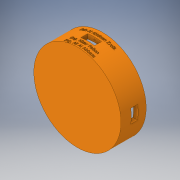
# Autodesk Inventor part: Base
Saved by Autodesk Inventor 2019 (Build 230136000, 136)
## iProperties
Created: 2022-07-05
Part Number: Base
Material: Generic
Document SubType Name: Modeling
Designer: zreik
Density: 1 g/cm^3
Appearance: Orange
Author: zreik
Autodesk Inventor part; units mm, degrees
(part 1 of 2)
ref_plane "YZ Plane" through (0, 0, 0) normal (1, 0, 0) x (0, 1, 0)
ref_plane "XY Plane" through (0, 0, 0) normal (0, 0, 1) x (1, 0, 0)
sketch "Sketch1" plane through (0, 0, 0) normal (0, 0, 1) x (1, 0, 0)
  circle A0 centre (0, 0) radius 95
  circle A1 centre (0, 0) radius 85
  circle A2 centre (0, 90) radius 1.5
  circle A3 centre (-77.9423, -45) radius 1.5
  circle A4 centre (77.9423, -45) radius 1.5
  dimension "d2" = 190
  dimension "d3" = 170
  dimension "d4" = 3
  dimension "d5" = 0
  dimension "d6" = 90
  dimension "d7" = 360
  constraints: 5 centre point, 3 coincident, 7 other
  measures "d2" diameter of A0
  measures "d3" diameter of A1
  measures "d4" diameter of A2
  measures "d5" horizontal distance of point (0, 0) A2.centre
  measures "d6" distance of point (0, 0) A2.centre
extrude "Extrusion1" add sketch "Sketch1" along normal blind 5 contours A0 | A1
extrude "Extrusion2" add sketch "Sketch1" against normal blind 50
extrude "Extrusion3" add sketch "Sketch1" along normal mid plane 10 contours A2 | A3 | A4
sketch "Sketch2" plane through (0, 0, 0) normal (0, 1, 0) x (-1, 0, 0)
  line L0 (-15, -17.5) -> (15, -17.5)
  line L1 (15, -17.5) -> (15, -32.5)
  line L2 (15, -32.5) -> (-15, -32.5)
  line L3 (-15, -32.5) -> (-15, -17.5)
  line L4 (-15, -17.5) -> (15, -32.5) construction
  line L5 (15, -17.5) -> (-15, -32.5) construction
  point P0 (0, 0)
  point P1 (0, -25)
  dimension "d14" = 0
  dimension "d15" = 25
  dimension "d16" = 30
  dimension "d17" = 15
  constraints: 12 end point, 2 midpoint, 2 parallel, 1 horizontal, 1 perpendicular
  measures "d14" horizontal distance of point (0, 0) point (0, -25)
  measures "d15" distance of point (0, 0) point (0, -25)
  measures "d16" distance of L1.end L2.end
  measures "d17" distance of L0.end L1.end
extrude "Extrusion4" cut sketch "Sketch2" against normal through all
pattern_circular "Circular Pattern1" count 4 over 360 about axis through (0, 0, 0) along (0, 0, -1) of "Extrusion4"
extrude "Extrusion5" add sketch "Sketch1" against normal blind 17.5 contours A2 | A3 | A4
ref_plane "Work Plane1" through (0, 100, 0) normal (0, 1, 0) x (-1, 0, 0)
sketch "Sketch3" plane through (0, 100, 0) normal (0, 1, 0) x (-1, 0, 0)
  line L0 (40, -45) -> (-40, -45) construction
  line L1 (-40, -45) -> (-40, -35) construction
  line L2 (-40, -35) -> (40, -35) construction
  line L3 (40, -35) -> (40, -45) construction
  line L4 (-95, -50) -> (95, -50) projected
  line L5 (40, -12.5) -> (-40, -12.5) construction
  line L6 (-40, -12.5) -> (-40, 2.5) construction
  line L7 (-40, 2.5) -> (40, 2.5) construction
  line L8 (40, 2.5) -> (40, -12.5) construction
  line L9 (95, 5) -> (-95, 5) projected
  line L10 (34.724, -36.8783) -> (38.9851, -36.8783)
  line L11 (38.9851, -36.8783) -> (38.9851, -37.6346)
  line L12 (38.9851, -37.6346) -> (35.7226, -42.2566)
  line L13 (35.7226, -42.2566) -> (38.8368, -42.2566)
  line L14 (38.8368, -42.2566) -> (38.8368, -42.9783)
  line L15 (38.8368, -42.9783) -> (34.8081, -42.9783)
  line L16 (34.8081, -42.9783) -> (34.8081, -42.2467)
  line L17 (34.8081, -42.2467) -> (38.1052, -37.6)
  line L18 (38.1052, -37.6) -> (34.724, -37.6)
  line L19 (34.724, -37.6) -> (34.724, -36.8783)
  spline S0 degree 2 poles (31.9953, -36.7745) (33.0927, -36.7745) (34.2989, -38.0054) (34.2989, -39.1423) knots 0 0 0 1 2 2 2
  spline S1 degree 2 poles (34.2989, -39.1423) (34.2989, -40.2595) (33.1274, -41.5843) (32.1832, -41.5843) knots 0 0 0 1 2 2 2
  spline S2 degree 2 poles (32.1832, -41.5843) (31.7581, -41.5843) (31.1006, -41.3372) (30.8584, -41.0752) knots 0 0 0 1 2 2 2
  spline S3 degree 2 poles (30.8584, -41.0752) (30.6112, -40.8132) (30.3492, -40.0568) (30.3492, -39.5081) knots 0 0 0 1 2 2 2
  line L20 (30.3492, -39.5081) -> (30.3492, -39.088)
  line L21 (30.3492, -39.088) -> (33.5179, -39.088)
  spline S4 degree 2 poles (33.5179, -39.088) (33.5179, -38.2921) (32.7171, -37.4468) (32.0052, -37.4468) knots 0 0 0 1 2 2 2
  spline S5 degree 2 poles (32.0052, -37.4468) (31.7531, -37.4468) (31.2637, -37.5605) (31.066, -37.6495) knots 0 0 0 1 2 2 2
  spline S6 degree 2 poles (31.066, -37.6495) (30.8584, -37.7483) (30.5717, -37.9214) (30.4778, -38.0004) knots 0 0 0 1 2 2 2
  line L22 (30.4778, -38.0004) -> (30.4333, -38.0004)
  line L23 (30.4333, -38.0004) -> (30.4333, -37.1601)
  spline S7 degree 2 poles (30.4333, -37.1601) (30.5667, -37.1057) (30.9721, -36.9475) (31.1303, -36.903) knots 0 0 0 1 2 2 2
  spline S8 degree 2 poles (31.1303, -36.903) (31.3527, -36.8388) (31.7185, -36.7745) (31.9953, -36.7745) knots 0 0 0 1 2 2 2
  spline S9 degree 2 poles (31.1006, -39.6762) (31.1105, -39.9876) (31.239, -40.4424) (31.3626, -40.5957) knots 0 0 0 1 2 2 2
  spline S10 degree 2 poles (31.3626, -40.5957) (31.4961, -40.7687) (31.9162, -40.9516) (32.2277, -40.9516) knots 0 0 0 1 2 2 2
  spline S11 degree 2 poles (32.2277, -40.9516) (32.5342, -40.9516) (32.9642, -40.7687) (33.1422, -40.5907) knots 0 0 0 1 2 2 2
  spline S12 degree 2 poles (33.1422, -40.5907) (33.3152, -40.4078) (33.4932, -39.9679) (33.5179, -39.6762) knots 0 0 0 1 2 2 2
  line L24 (33.5179, -39.6762) -> (31.1006, -39.6762)
  line L25 (28.7822, -36.8783) -> (29.5534, -36.8783)
  line L26 (29.5534, -36.8783) -> (29.5534, -41.4558)
  line L27 (29.5534, -41.4558) -> (28.7822, -41.4558)
  line L28 (28.7822, -41.4558) -> (28.7822, -36.8783)
  line L29 (28.7278, -42.2171) -> (29.6028, -42.2171)
  line L30 (29.6028, -42.2171) -> (29.6028, -43.0179)
  line L31 (29.6028, -43.0179) -> (28.7278, -43.0179)
  line L32 (28.7278, -43.0179) -> (28.7278, -42.2171)
  line L33 (24.0564, -36.8783) -> (24.8276, -36.8783)
  line L34 (24.8276, -36.8783) -> (24.8276, -39.4884)
  spline S13 degree 2 poles (24.8276, -39.4884) (24.8276, -39.8047) (24.8869, -40.3485) (24.9759, -40.5116) knots 0 0 0 1 2 2 2
  spline S14 degree 2 poles (24.9759, -40.5116) (25.0698, -40.6846) (25.406, -40.8527) (25.6927, -40.8527) knots 0 0 0 1 2 2 2
  spline S15 degree 2 poles (25.6927, -40.8527) (25.9794, -40.8527) (26.5874, -40.5462) (26.8791, -40.2991) knots 0 0 0 1 2 2 2
  line L35 (26.8791, -40.2991) -> (26.8791, -36.8783)
  line L36 (26.8791, -36.8783) -> (27.6502, -36.8783)
  line L37 (27.6502, -36.8783) -> (27.6502, -41.4558)
  line L38 (27.6502, -41.4558) -> (26.8791, -41.4558)
  line L39 (26.8791, -41.4558) -> (26.8791, -40.9466)
  spline S16 degree 2 poles (26.8791, -40.9466) (26.533, -41.2581) (25.8657, -41.5843) (25.49, -41.5843) knots 0 0 0 1 2 2 2
  spline S17 degree 2 poles (25.49, -41.5843) (24.8177, -41.5843) (24.0564, -40.6945) (24.0564, -39.8492) knots 0 0 0 1 2 2 2
  line L40 (24.0564, -39.8492) -> (24.0564, -36.8783)
  line L41 (20.9521, -36.8783) -> (18.8957, -42.9783)
  line L42 (18.8957, -42.9783) -> (17.8971, -42.9783)
  line L43 (17.8971, -42.9783) -> (15.8407, -36.8783)
  line L44 (15.8407, -36.8783) -> (16.6959, -36.8783)
  line L45 (16.6959, -36.8783) -> (17.2496, -38.5838)
  line L46 (17.2496, -38.5838) -> (19.5778, -38.5838)
  line L47 (19.5778, -38.5838) -> (20.1315, -36.8783)
  line L48 (20.1315, -36.8783) -> (20.9521, -36.8783)
  line L49 (17.472, -39.2758) -> (18.4162, -42.1479)
  line L50 (18.4162, -42.1479) -> (19.3554, -39.2758)
  line L51 (19.3554, -39.2758) -> (17.472, -39.2758)
  line L52 (14.5357, -36.8783) -> (15.3068, -36.8783)
  line L53 (15.3068, -36.8783) -> (15.3068, -43.2502)
  line L54 (15.3068, -43.2502) -> (14.5357, -43.2502)
  line L55 (14.5357, -43.2502) -> (14.5357, -36.8783)
  line L56 (11.3819, -36.8783) -> (9.3255, -42.9783)
  line L57 (9.3255, -42.9783) -> (8.3269, -42.9783)
  line L58 (8.3269, -42.9783) -> (6.2705, -36.8783)
  line L59 (6.2705, -36.8783) -> (7.1257, -36.8783)
  line L60 (7.1257, -36.8783) -> (7.6794, -38.5838)
  line L61 (7.6794, -38.5838) -> (10.0077, -38.5838)
  line L62 (10.0077, -38.5838) -> (10.5613, -36.8783)
  line L63 (10.5613, -36.8783) -> (11.3819, -36.8783)
  line L64 (7.9018, -39.2758) -> (8.846, -42.1479)
  line L65 (8.846, -42.1479) -> (9.7852, -39.2758)
  line L66 (9.7852, -39.2758) -> (7.9018, -39.2758)
  spline S18 degree 2 poles (1.9155, -39.2412) (1.9155, -38.1191) (3.003, -36.7498) (3.8236, -36.7498) knots 0 0 0 1 2 2 2
  spline S19 degree 2 poles (3.8236, -36.7498) (4.1944, -36.7498) (4.7233, -36.9327) (4.9803, -37.0909) knots 0 0 0 1 2 2 2
  line L67 (4.9803, -37.0909) -> (5.0298, -36.8783)
  line L68 (5.0298, -36.8783) -> (5.7515, -36.8783)
  line L69 (5.7515, -36.8783) -> (5.7515, -43.2502)
  line L70 (5.7515, -43.2502) -> (4.9803, -43.2502)
  line L71 (4.9803, -43.2502) -> (4.9803, -40.9763)
  spline S20 degree 2 poles (4.9803, -40.9763) (4.6887, -41.2383) (4.0115, -41.5843) (3.5814, -41.5843) knots 0 0 0 1 2 2 2
  spline S21 degree 2 poles (3.5814, -41.5843) (2.8053, -41.5843) (1.9155, -40.3436) (1.9155, -39.2412) knots 0 0 0 1 2 2 2
  spline S22 degree 2 poles (2.7114, -39.1819) (2.7114, -40.0025) (3.2107, -40.8527) (3.7643, -40.8527) knots 0 0 0 1 2 2 2
  spline S23 degree 2 poles (3.7643, -40.8527) (4.0757, -40.8527) (4.7184, -40.5561) (4.9803, -40.3287) knots 0 0 0 1 2 2 2
  line L72 (4.9803, -40.3287) -> (4.9803, -37.7038)
  spline S24 degree 2 poles (4.9803, -37.7038) (4.6887, -37.5605) (4.2389, -37.4419) (3.9719, -37.4419) knots 0 0 0 1 2 2 2
  spline S25 degree 2 poles (3.9719, -37.4419) (3.3837, -37.4419) (2.7114, -38.2773) (2.7114, -39.1819) knots 0 0 0 1 2 2 2
  line L73 (0.3287, -36.8783) -> (1.0999, -36.8783)
  line L74 (1.0999, -36.8783) -> (1.0999, -41.4558)
  line L75 (1.0999, -41.4558) -> (0.3287, -41.4558)
  line L76 (0.3287, -41.4558) -> (0.3287, -36.8783)
  line L77 (0.2744, -42.2171) -> (1.1493, -42.2171)
  line L78 (1.1493, -42.2171) -> (1.1493, -43.0179)
  line L79 (1.1493, -43.0179) -> (0.2744, -43.0179)
  line L80 (0.2744, -43.0179) -> (0.2744, -42.2171)
  line L81 (-4.3229, -36.8783) -> (-3.5517, -36.8783)
  line L82 (-3.5517, -36.8783) -> (-3.5517, -37.343)
  spline S26 degree 2 poles (-3.5517, -37.343) (-3.3738, -37.1947) (-3.1118, -36.997) (-2.9338, -36.9129) knots 0 0 0 1 2 2 2
  spline S27 degree 2 poles (-2.9338, -36.9129) (-2.7707, -36.8338) (-2.4197, -36.7498) (-2.1874, -36.7498) knots 0 0 0 1 2 2 2
  spline S28 degree 2 poles (-2.1874, -36.7498) (-1.8117, -36.7498) (-1.179, -37.0612) (-0.9565, -37.3628) knots 0 0 0 1 2 2 2
  spline S29 degree 2 poles (-0.9565, -37.3628) (-0.7341, -37.6643) (-0.4869, -38.5541) (-0.4869, -39.1325) knots 0 0 0 1 2 2 2
  spline S30 degree 2 poles (-0.4869, -39.1325) (-0.4869, -39.7355) (-0.7983, -40.6154) (-1.0702, -40.9466) knots 0 0 0 1 2 2 2
  spline S31 degree 2 poles (-1.0702, -40.9466) (-1.3223, -41.2432) (-2.0292, -41.5843) (-2.4197, -41.5843) knots 0 0 0 1 2 2 2
  spline S32 degree 2 poles (-2.4197, -41.5843) (-2.7608, -41.5843) (-3.27, -41.4311) (-3.5517, -41.2729) knots 0 0 0 1 2 2 2
  line L83 (-3.5517, -41.2729) -> (-3.5517, -43.2502)
  line L84 (-3.5517, -43.2502) -> (-4.3229, -43.2502)
  line L85 (-4.3229, -43.2502) -> (-4.3229, -36.8783)
  line L86 (-3.5517, -37.9906) -> (-3.5517, -40.6352)
  spline S33 degree 2 poles (-3.5517, -40.6352) (-3.265, -40.7736) (-2.8103, -40.8774) (-2.5483, -40.8774) knots 0 0 0 1 2 2 2
  spline S34 degree 2 poles (-2.5483, -40.8774) (-1.9551, -40.8774) (-1.2828, -39.9876) (-1.2828, -39.1473) knots 0 0 0 1 2 2 2
  spline S35 degree 2 poles (-1.2828, -39.1473) (-1.2828, -38.3366) (-1.7969, -37.4814) (-2.3654, -37.4814) knots 0 0 0 1 2 2 2
  spline S36 degree 2 poles (-2.3654, -37.4814) (-2.6669, -37.4814) (-3.2799, -37.7582) (-3.5517, -37.9906) knots 0 0 0 1 2 2 2
  spline S37 degree 2 poles (-7.4273, -36.7745) (-6.3299, -36.7745) (-5.1237, -38.0054) (-5.1237, -39.1423) knots 0 0 0 1 2 2 2
  spline S38 degree 2 poles (-5.1237, -39.1423) (-5.1237, -40.2595) (-6.2953, -41.5843) (-7.2394, -41.5843) knots 0 0 0 1 2 2 2
  spline S39 degree 2 poles (-7.2394, -41.5843) (-7.6645, -41.5843) (-8.322, -41.3372) (-8.5642, -41.0752) knots 0 0 0 1 2 2 2
  spline S40 degree 2 poles (-8.5642, -41.0752) (-8.8114, -40.8132) (-9.0734, -40.0568) (-9.0734, -39.5081) knots 0 0 0 1 2 2 2
  line L87 (-9.0734, -39.5081) -> (-9.0734, -39.088)
  line L88 (-9.0734, -39.088) -> (-5.9047, -39.088)
  spline S41 degree 2 poles (-5.9047, -39.088) (-5.9047, -38.2921) (-6.7056, -37.4468) (-7.4174, -37.4468) knots 0 0 0 1 2 2 2
  spline S42 degree 2 poles (-7.4174, -37.4468) (-7.6695, -37.4468) (-8.1589, -37.5605) (-8.3566, -37.6495) knots 0 0 0 1 2 2 2
  spline S43 degree 2 poles (-8.3566, -37.6495) (-8.5642, -37.7483) (-8.8509, -37.9214) (-8.9449, -38.0004) knots 0 0 0 1 2 2 2
  line L89 (-8.9449, -38.0004) -> (-8.9893, -38.0004)
  line L90 (-8.9893, -38.0004) -> (-8.9893, -37.1601)
  spline S44 degree 2 poles (-8.9893, -37.1601) (-8.8559, -37.1057) (-8.4505, -36.9475) (-8.2923, -36.903) knots 0 0 0 1 2 2 2
  spline S45 degree 2 poles (-8.2923, -36.903) (-8.0699, -36.8388) (-7.7041, -36.7745) (-7.4273, -36.7745) knots 0 0 0 1 2 2 2
  spline S46 degree 2 poles (-8.322, -39.6762) (-8.3121, -39.9876) (-8.1836, -40.4424) (-8.06, -40.5957) knots 0 0 0 1 2 2 2
  spline S47 degree 2 poles (-8.06, -40.5957) (-7.9265, -40.7687) (-7.5064, -40.9516) (-7.1949, -40.9516) knots 0 0 0 1 2 2 2
  spline S48 degree 2 poles (-7.1949, -40.9516) (-6.8885, -40.9516) (-6.4584, -40.7687) (-6.2804, -40.5907) knots 0 0 0 1 2 2 2
  spline S49 degree 2 poles (-6.2804, -40.5907) (-6.1074, -40.4078) (-5.9295, -39.9679) (-5.9047, -39.6762) knots 0 0 0 1 2 2 2
  line L91 (-5.9047, -39.6762) -> (-8.322, -39.6762)
  spline S50 degree 2 poles (-11.8416, -36.7745) (-10.7442, -36.7745) (-9.538, -38.0054) (-9.538, -39.1423) knots 0 0 0 1 2 2 2
  spline S51 degree 2 poles (-9.538, -39.1423) (-9.538, -40.2595) (-10.7096, -41.5843) (-11.6538, -41.5843) knots 0 0 0 1 2 2 2
  spline S52 degree 2 poles (-11.6538, -41.5843) (-12.0789, -41.5843) (-12.7363, -41.3372) (-12.9786, -41.0752) knots 0 0 0 1 2 2 2
  spline S53 degree 2 poles (-12.9786, -41.0752) (-13.2257, -40.8132) (-13.4877, -40.0568) (-13.4877, -39.5081) knots 0 0 0 1 2 2 2
  line L92 (-13.4877, -39.5081) -> (-13.4877, -39.088)
  line L93 (-13.4877, -39.088) -> (-10.3191, -39.088)
  spline S54 degree 2 poles (-10.3191, -39.088) (-10.3191, -38.2921) (-11.1199, -37.4468) (-11.8317, -37.4468) knots 0 0 0 1 2 2 2
  spline S55 degree 2 poles (-11.8317, -37.4468) (-12.0838, -37.4468) (-12.5732, -37.5605) (-12.7709, -37.6495) knots 0 0 0 1 2 2 2
  spline S56 degree 2 poles (-12.7709, -37.6495) (-12.9786, -37.7483) (-13.2653, -37.9214) (-13.3592, -38.0004) knots 0 0 0 1 2 2 2
  line L94 (-13.3592, -38.0004) -> (-13.4037, -38.0004)
  line L95 (-13.4037, -38.0004) -> (-13.4037, -37.1601)
  spline S57 degree 2 poles (-13.4037, -37.1601) (-13.2702, -37.1057) (-12.8649, -36.9475) (-12.7067, -36.903) knots 0 0 0 1 2 2 2
  spline S58 degree 2 poles (-12.7067, -36.903) (-12.4842, -36.8388) (-12.1184, -36.7745) (-11.8416, -36.7745) knots 0 0 0 1 2 2 2
  spline S59 degree 2 poles (-12.7363, -39.6762) (-12.7265, -39.9876) (-12.5979, -40.4424) (-12.4744, -40.5957) knots 0 0 0 1 2 2 2
  spline S60 degree 2 poles (-12.4744, -40.5957) (-12.3409, -40.7687) (-11.9207, -40.9516) (-11.6093, -40.9516) knots 0 0 0 1 2 2 2
  spline S61 degree 2 poles (-11.6093, -40.9516) (-11.3028, -40.9516) (-10.8727, -40.7687) (-10.6948, -40.5907) knots 0 0 0 1 2 2 2
  spline S62 degree 2 poles (-10.6948, -40.5907) (-10.5218, -40.4078) (-10.3438, -39.9679) (-10.3191, -39.6762) knots 0 0 0 1 2 2 2
  line L96 (-10.3191, -39.6762) -> (-12.7363, -39.6762)
  line L97 (-17.8625, -36.8783) -> (-17.0914, -36.8783)
  line L98 (-17.0914, -36.8783) -> (-17.0914, -39.4884)
  spline S63 degree 2 poles (-17.0914, -39.4884) (-17.0914, -39.8047) (-17.0321, -40.3485) (-16.9431, -40.5116) knots 0 0 0 1 2 2 2
  spline S64 degree 2 poles (-16.9431, -40.5116) (-16.8491, -40.6846) (-16.513, -40.8527) (-16.2263, -40.8527) knots 0 0 0 1 2 2 2
  spline S65 degree 2 poles (-16.2263, -40.8527) (-15.9396, -40.8527) (-15.3316, -40.5462) (-15.0399, -40.2991) knots 0 0 0 1 2 2 2
  line L99 (-15.0399, -40.2991) -> (-15.0399, -36.8783)
  line L100 (-15.0399, -36.8783) -> (-14.2688, -36.8783)
  line L101 (-14.2688, -36.8783) -> (-14.2688, -41.4558)
  line L102 (-14.2688, -41.4558) -> (-15.0399, -41.4558)
  line L103 (-15.0399, -41.4558) -> (-15.0399, -40.9466)
  spline S66 degree 2 poles (-15.0399, -40.9466) (-15.3859, -41.2581) (-16.0533, -41.5843) (-16.429, -41.5843) knots 0 0 0 1 2 2 2
  spline S67 degree 2 poles (-16.429, -41.5843) (-17.1013, -41.5843) (-17.8625, -40.6945) (-17.8625, -39.8492) knots 0 0 0 1 2 2 2
  line L104 (-17.8625, -39.8492) -> (-17.8625, -36.8783)
  line L105 (-25.5147, -36.8783) -> (-21.2536, -36.8783)
  line L106 (-21.2536, -36.8783) -> (-21.2536, -37.6346)
  line L107 (-21.2536, -37.6346) -> (-24.5162, -42.2566)
  line L108 (-24.5162, -42.2566) -> (-21.4019, -42.2566)
  line L109 (-21.4019, -42.2566) -> (-21.4019, -42.9783)
  line L110 (-21.4019, -42.9783) -> (-25.4307, -42.9783)
  line L111 (-25.4307, -42.9783) -> (-25.4307, -42.2467)
  line L112 (-25.4307, -42.2467) -> (-22.1335, -37.6)
  line L113 (-22.1335, -37.6) -> (-25.5147, -37.6)
  line L114 (-25.5147, -37.6) -> (-25.5147, -36.8783)
  line L115 (-28.6833, -40.6303) -> (-28.6438, -40.6303)
  spline S68 degree 2 poles (-28.6438, -40.6303) (-28.5548, -40.655) (-28.362, -40.6649) (-28.2286, -40.6649) knots 0 0 0 1 2 2 2
  spline S69 degree 2 poles (-28.2286, -40.6649) (-27.9171, -40.6649) (-27.3042, -40.393) (-27.0274, -40.1261) knots 0 0 0 1 2 2 2
  line L116 (-27.0274, -40.1261) -> (-27.0274, -36.8783)
  line L117 (-27.0274, -36.8783) -> (-26.2562, -36.8783)
  line L118 (-26.2562, -36.8783) -> (-26.2562, -41.4558)
  line L119 (-26.2562, -41.4558) -> (-27.0274, -41.4558)
  line L120 (-27.0274, -41.4558) -> (-27.0274, -40.7736)
  spline S70 degree 2 poles (-27.0274, -40.7736) (-27.4475, -41.1493) (-28.0753, -41.4558) (-28.3719, -41.4558) knots 0 0 0 1 2 2 2
  spline S71 degree 2 poles (-28.3719, -41.4558) (-28.4906, -41.4558) (-28.6092, -41.4459) (-28.6833, -41.4311) knots 0 0 0 1 2 2 2
  line L121 (-28.6833, -41.4311) -> (-28.6833, -40.6303)
  spline S72 degree 2 poles (-31.2687, -36.7745) (-30.1713, -36.7745) (-28.9651, -38.0054) (-28.9651, -39.1423) knots 0 0 0 1 2 2 2
  spline S73 degree 2 poles (-28.9651, -39.1423) (-28.9651, -40.2595) (-30.1367, -41.5843) (-31.0808, -41.5843) knots 0 0 0 1 2 2 2
  spline S74 degree 2 poles (-31.0808, -41.5843) (-31.506, -41.5843) (-32.1634, -41.3372) (-32.4056, -41.0752) knots 0 0 0 1 2 2 2
  spline S75 degree 2 poles (-32.4056, -41.0752) (-32.6528, -40.8132) (-32.9148, -40.0568) (-32.9148, -39.5081) knots 0 0 0 1 2 2 2
  line L122 (-32.9148, -39.5081) -> (-32.9148, -39.088)
  line L123 (-32.9148, -39.088) -> (-29.7462, -39.088)
  spline S76 degree 2 poles (-29.7462, -39.088) (-29.7462, -38.2921) (-30.547, -37.4468) (-31.2588, -37.4468) knots 0 0 0 1 2 2 2
  spline S77 degree 2 poles (-31.2588, -37.4468) (-31.5109, -37.4468) (-32.0003, -37.5605) (-32.198, -37.6495) knots 0 0 0 1 2 2 2
  spline S78 degree 2 poles (-32.198, -37.6495) (-32.4056, -37.7483) (-32.6923, -37.9214) (-32.7863, -38.0004) knots 0 0 0 1 2 2 2
  line L124 (-32.7863, -38.0004) -> (-32.8308, -38.0004)
  line L125 (-32.8308, -38.0004) -> (-32.8308, -37.1601)
  spline S79 degree 2 poles (-32.8308, -37.1601) (-32.6973, -37.1057) (-32.2919, -36.9475) (-32.1338, -36.903) knots 0 0 0 1 2 2 2
  spline S80 degree 2 poles (-32.1338, -36.903) (-31.9113, -36.8388) (-31.5455, -36.7745) (-31.2687, -36.7745) knots 0 0 0 1 2 2 2
  spline S81 degree 2 poles (-32.1634, -39.6762) (-32.1535, -39.9876) (-32.025, -40.4424) (-31.9014, -40.5957) knots 0 0 0 1 2 2 2
  spline S82 degree 2 poles (-31.9014, -40.5957) (-31.768, -40.7687) (-31.3478, -40.9516) (-31.0363, -40.9516) knots 0 0 0 1 2 2 2
  spline S83 degree 2 poles (-31.0363, -40.9516) (-30.7299, -40.9516) (-30.2998, -40.7687) (-30.1218, -40.5907) knots 0 0 0 1 2 2 2
  spline S84 degree 2 poles (-30.1218, -40.5907) (-29.9488, -40.4078) (-29.7709, -39.9679) (-29.7462, -39.6762) knots 0 0 0 1 2 2 2
  line L126 (-29.7462, -39.6762) -> (-32.1634, -39.6762)
  line L127 (-34.4818, -36.8783) -> (-33.7107, -36.8783)
  line L128 (-33.7107, -36.8783) -> (-33.7107, -41.4558)
  line L129 (-33.7107, -41.4558) -> (-34.4818, -41.4558)
  line L130 (-34.4818, -41.4558) -> (-34.4818, -36.8783)
  line L131 (-34.5362, -42.2171) -> (-33.6612, -42.2171)
  line L132 (-33.6612, -42.2171) -> (-33.6612, -43.0179)
  line L133 (-33.6612, -43.0179) -> (-34.5362, -43.0179)
  line L134 (-34.5362, -43.0179) -> (-34.5362, -42.2171)
  line L135 (-39.4053, -36.8783) -> (-38.3919, -36.8783)
  line L136 (-38.3919, -36.8783) -> (-36.6915, -39.088)
  line L137 (-36.6915, -39.088) -> (-36.385, -38.7914)
  line L138 (-36.385, -38.7914) -> (-36.385, -36.8783)
  line L139 (-36.385, -36.8783) -> (-35.6138, -36.8783)
  line L140 (-35.6138, -36.8783) -> (-35.6138, -43.2502)
  line L141 (-35.6138, -43.2502) -> (-36.385, -43.2502)
  line L142 (-36.385, -43.2502) -> (-36.385, -39.523)
  line L143 (-36.385, -39.523) -> (-38.1942, -41.4558)
  line L144 (-38.1942, -41.4558) -> (-39.1532, -41.4558)
  line L145 (-39.1532, -41.4558) -> (-37.2748, -39.5427)
  line L146 (-37.2748, -39.5427) -> (-39.4053, -36.8783)
  line L147 (30.542, -7.7009) -> (30.542, -13.8009)
  line L148 (30.542, -13.8009) -> (26.7258, -13.8009)
  line L149 (26.7258, -13.8009) -> (26.7258, -13.0792)
  line L150 (26.7258, -13.0792) -> (29.7313, -13.0792)
  line L151 (29.7313, -13.0792) -> (29.7313, -11.4083)
  line L152 (29.7313, -11.4083) -> (26.9285, -11.4083)
  line L153 (26.9285, -11.4083) -> (26.9285, -10.6866)
  line L154 (26.9285, -10.6866) -> (29.7313, -10.6866)
  line L155 (29.7313, -10.6866) -> (29.7313, -8.4226)
  line L156 (29.7313, -8.4226) -> (26.7258, -8.4226)
  line L157 (26.7258, -8.4226) -> (26.7258, -7.7009)
  line L158 (26.7258, -7.7009) -> (30.542, -7.7009)
  line L159 (22.3016, -7.7009) -> (23.0727, -7.7009)
  line L160 (23.0727, -7.7009) -> (23.0727, -10.3109)
  spline S85 degree 2 poles (23.0727, -10.3109) (23.0727, -10.6273) (23.1321, -11.1711) (23.221, -11.3342) knots 0 0 0 1 2 2 2
  spline S86 degree 2 poles (23.221, -11.3342) (23.315, -11.5072) (23.6511, -11.6753) (23.9378, -11.6753) knots 0 0 0 1 2 2 2
  spline S87 degree 2 poles (23.9378, -11.6753) (24.2245, -11.6753) (24.8325, -11.3688) (25.1242, -11.1216) knots 0 0 0 1 2 2 2
  line L161 (25.1242, -11.1216) -> (25.1242, -7.7009)
  line L162 (25.1242, -7.7009) -> (25.8953, -7.7009)
  line L163 (25.8953, -7.7009) -> (25.8953, -12.2783)
  line L164 (25.8953, -12.2783) -> (25.1242, -12.2783)
  line L165 (25.1242, -12.2783) -> (25.1242, -11.7692)
  spline S88 degree 2 poles (25.1242, -11.7692) (24.7782, -12.0806) (24.1108, -12.4069) (23.7351, -12.4069) knots 0 0 0 1 2 2 2
  spline S89 degree 2 poles (23.7351, -12.4069) (23.0628, -12.4069) (22.3016, -11.5171) (22.3016, -10.6718) knots 0 0 0 1 2 2 2
  line L166 (22.3016, -10.6718) -> (22.3016, -7.7009)
  spline S90 degree 2 poles (21.0559, -6.9693) (20.9768, -6.9347) (20.6752, -6.8259) (20.4825, -6.7814) knots 0 0 0 1 2 2 2
  spline S91 degree 2 poles (20.4825, -6.7814) (20.2699, -6.7271) (19.909, -6.6628) (19.6965, -6.6628) knots 0 0 0 1 2 2 2
  spline S92 degree 2 poles (19.6965, -6.6628) (19.3406, -6.6628) (18.8462, -6.8506) (18.7078, -7.0187) knots 0 0 0 1 2 2 2
  spline S93 degree 2 poles (18.7078, -7.0187) (18.5744, -7.1868) (18.4705, -7.6267) (18.4705, -7.9085) knots 0 0 0 1 2 2 2
  line L167 (18.4705, -7.9085) -> (18.4705, -8.3089)
  spline S94 degree 2 poles (18.4705, -8.3089) (18.782, -8.037) (19.3801, -7.78) (19.8299, -7.78) knots 0 0 0 1 2 2 2
  spline S95 degree 2 poles (19.8299, -7.78) (20.611, -7.78) (21.5354, -8.9416) (21.5354, -10.0341) knots 0 0 0 1 2 2 2
  spline S96 degree 2 poles (21.5354, -10.0341) (21.5354, -10.6026) (21.2141, -11.4825) (20.9471, -11.7939) knots 0 0 0 1 2 2 2
  spline S97 degree 2 poles (20.9471, -11.7939) (20.6901, -12.0856) (19.9832, -12.4069) (19.6075, -12.4069) knots 0 0 0 1 2 2 2
  spline S98 degree 2 poles (19.6075, -12.4069) (19.2516, -12.4069) (18.7325, -12.2388) (18.4705, -12.0856) knots 0 0 0 1 2 2 2
  line L168 (18.4705, -12.0856) -> (18.4261, -12.2783)
  line L169 (18.4261, -12.2783) -> (17.6994, -12.2783)
  line L170 (17.6994, -12.2783) -> (17.6994, -8.2249)
  spline S99 degree 2 poles (17.6994, -8.2249) (17.6994, -7.0583) (18.7128, -5.9707) (19.7558, -5.9707) knots 0 0 0 1 2 2 2
  spline S100 degree 2 poles (19.7558, -5.9707) (20.0919, -5.9707) (20.7939, -6.0795) (21.0954, -6.1685) knots 0 0 0 1 2 2 2
  line L171 (21.0954, -6.1685) -> (21.0954, -6.9693)
  line L172 (21.0954, -6.9693) -> (21.0559, -6.9693)
  line L173 (18.4705, -8.9416) -> (18.4705, -11.4578)
  spline S101 degree 2 poles (18.4705, -11.4578) (18.7573, -11.5962) (19.2417, -11.7148) (19.4839, -11.7148) knots 0 0 0 1 2 2 2
  spline S102 degree 2 poles (19.4839, -11.7148) (20.0672, -11.7148) (20.7395, -10.8547) (20.7395, -10.0489) knots 0 0 0 1 2 2 2
  spline S103 degree 2 poles (20.7395, -10.0489) (20.7395, -9.2877) (20.2303, -8.4918) (19.6569, -8.4918) knots 0 0 0 1 2 2 2
  spline S104 degree 2 poles (19.6569, -8.4918) (19.3554, -8.4918) (18.7227, -8.7291) (18.4705, -8.9416) knots 0 0 0 1 2 2 2
  line L174 (15.3859, -7.7009) -> (16.3647, -7.7009)
  line L175 (16.3647, -7.7009) -> (16.3647, -8.8675)
  line L176 (16.3647, -8.8675) -> (15.3859, -8.8675)
  line L177 (15.3859, -8.8675) -> (15.3859, -7.7009)
  line L178 (6.9972, -7.7009) -> (7.9068, -7.7009)
  line L179 (7.9068, -7.7009) -> (10.6058, -12.9605)
  line L180 (10.6058, -12.9605) -> (10.6058, -7.7009)
  line L181 (10.6058, -7.7009) -> (11.3621, -7.7009)
  line L182 (11.3621, -7.7009) -> (11.3621, -13.8009)
  line L183 (11.3621, -13.8009) -> (10.2103, -13.8009)
  line L184 (10.2103, -13.8009) -> (7.7535, -8.9713)
  line L185 (7.7535, -8.9713) -> (7.7535, -13.8009)
  line L186 (7.7535, -13.8009) -> (6.9972, -13.8009)
  line L187 (6.9972, -13.8009) -> (6.9972, -7.7009)
  line L188 (5.0347, -7.7009) -> (5.8059, -7.7009)
  line L189 (5.8059, -7.7009) -> (5.8059, -12.2783)
  line L190 (5.8059, -12.2783) -> (5.0347, -12.2783)
  line L191 (5.0347, -12.2783) -> (5.0347, -7.7009)
  line L192 (4.9803, -13.0396) -> (5.8553, -13.0396)
  line L193 (5.8553, -13.0396) -> (5.8553, -13.8404)
  line L194 (5.8553, -13.8404) -> (4.9803, -13.8404)
  line L195 (4.9803, -13.8404) -> (4.9803, -13.0396)
  line L196 (0.8972, -7.7009) -> (4.2586, -7.7009)
  line L197 (4.2586, -7.7009) -> (4.2586, -8.2743)
  line L198 (4.2586, -8.2743) -> (1.8661, -11.6456)
  line L199 (1.8661, -11.6456) -> (4.1598, -11.6456)
  line L200 (4.1598, -11.6456) -> (4.1598, -12.2783)
  line L201 (4.1598, -12.2783) -> (0.9417, -12.2783)
  line L202 (0.9417, -12.2783) -> (0.9417, -11.7296)
  line L203 (0.9417, -11.7296) -> (3.3441, -8.3484)
  line L204 (3.3441, -8.3484) -> (0.8972, -8.3484)
  line L205 (0.8972, -8.3484) -> (0.8972, -7.7009)
  spline S105 degree 2 poles (-2.3752, -8.1853) (-2.2813, -8.1161) (-1.965, -7.8689) (-1.8167, -7.7948) knots 0 0 0 1 2 2 2
  spline S106 degree 2 poles (-1.8167, -7.7948) (-1.614, -7.686) (-1.2333, -7.5724) (-0.8873, -7.5724) knots 0 0 0 1 2 2 2
  spline S107 degree 2 poles (-0.8873, -7.5724) (-0.6056, -7.5724) (-0.0964, -7.7849) (0.0964, -7.9777) knots 0 0 0 1 2 2 2
  spline S108 degree 2 poles (0.0964, -7.9777) (0.2793, -8.1655) (0.5017, -8.7192) (0.5017, -9.0257) knots 0 0 0 1 2 2 2
  spline S109 degree 2 poles (0.5017, -9.0257) (0.5017, -9.5002) (0.1013, -10.1725) (-0.3337, -10.3653) knots 0 0 0 1 2 2 2
  spline S110 degree 2 poles (-0.3337, -10.3653) (-0.7192, -10.5433) (-1.7672, -10.6767) (-2.3752, -10.7113) knots 0 0 0 1 2 2 2
  line L206 (-2.3752, -10.7113) -> (-2.3752, -10.8596)
  spline S111 degree 2 poles (-2.3752, -10.8596) (-2.3752, -11.1266) (-2.2121, -11.4578) (-2.0638, -11.5517) knots 0 0 0 1 2 2 2
  spline S112 degree 2 poles (-2.0638, -11.5517) (-1.9155, -11.6456) (-1.4904, -11.7049) (-1.263, -11.7049) knots 0 0 0 1 2 2 2
  spline S113 degree 2 poles (-1.263, -11.7049) (-0.9961, -11.7049) (-0.2744, -11.5467) (0.0865, -11.3935) knots 0 0 0 1 2 2 2
  line L207 (0.0865, -11.3935) -> (0.131, -11.3935)
  line L208 (0.131, -11.3935) -> (0.131, -12.1795)
  spline S114 degree 2 poles (0.131, -12.1795) (-0.0816, -12.2388) (-0.8774, -12.3871) (-1.2679, -12.3871) knots 0 0 0 1 2 2 2
  spline S115 degree 2 poles (-1.2679, -12.3871) (-1.7425, -12.3871) (-2.3901, -12.2388) (-2.6471, -12.046) knots 0 0 0 1 2 2 2
  spline S116 degree 2 poles (-2.6471, -12.046) (-2.8992, -11.8582) (-3.1464, -11.26) (-3.1464, -10.83) knots 0 0 0 1 2 2 2
  line L209 (-3.1464, -10.83) -> (-3.1464, -7.7009)
  line L210 (-3.1464, -7.7009) -> (-2.3752, -7.7009)
  line L211 (-2.3752, -7.7009) -> (-2.3752, -8.1853)
  line L212 (-2.3752, -8.8279) -> (-2.3752, -10.0984)
  spline S117 degree 2 poles (-2.3752, -10.0984) (-2.0984, -10.0736) (-1.263, -9.9896) (-1.001, -9.9105) knots 0 0 0 1 2 2 2
  spline S118 degree 2 poles (-1.001, -9.9105) (-0.6945, -9.8166) (-0.2941, -9.4261) (-0.2941, -9.0801) knots 0 0 0 1 2 2 2
  spline S119 degree 2 poles (-0.2941, -9.0801) (-0.2941, -8.6846) (-0.739, -8.2842) (-1.1641, -8.2842) knots 0 0 0 1 2 2 2
  spline S120 degree 2 poles (-1.1641, -8.2842) (-1.525, -8.2842) (-2.1182, -8.5956) (-2.3752, -8.8279) knots 0 0 0 1 2 2 2
  line L213 (-6.6561, -11.4528) -> (-6.6166, -11.4528)
  spline S121 degree 2 poles (-6.6166, -11.4528) (-6.5276, -11.4775) (-6.3348, -11.4874) (-6.2013, -11.4874) knots 0 0 0 1 2 2 2
  spline S122 degree 2 poles (-6.2013, -11.4874) (-5.8899, -11.4874) (-5.2769, -11.2155) (-5.0001, -10.9486) knots 0 0 0 1 2 2 2
  line L214 (-5.0001, -10.9486) -> (-5.0001, -7.7009)
  line L215 (-5.0001, -7.7009) -> (-4.229, -7.7009)
  line L216 (-4.229, -7.7009) -> (-4.229, -12.2783)
  line L217 (-4.229, -12.2783) -> (-5.0001, -12.2783)
  line L218 (-5.0001, -12.2783) -> (-5.0001, -11.5962)
  spline S123 degree 2 poles (-5.0001, -11.5962) (-5.4203, -11.9719) (-6.0481, -12.2783) (-6.3447, -12.2783) knots 0 0 0 1 2 2 2
  spline S124 degree 2 poles (-6.3447, -12.2783) (-6.4633, -12.2783) (-6.582, -12.2685) (-6.6561, -12.2536) knots 0 0 0 1 2 2 2
  line L219 (-6.6561, -12.2536) -> (-6.6561, -11.4528)
  line L220 (-13.5816, -13.0792) -> (-10.7442, -13.0792)
  line L221 (-10.7442, -13.0792) -> (-10.7442, -11.3589)
  line L222 (-10.7442, -11.3589) -> (-13.463, -11.3589)
  line L223 (-13.463, -11.3589) -> (-13.463, -10.6372)
  line L224 (-13.463, -10.6372) -> (-10.7442, -10.6372)
  line L225 (-10.7442, -10.6372) -> (-10.7442, -7.7009)
  line L226 (-10.7442, -7.7009) -> (-9.9335, -7.7009)
  line L227 (-9.9335, -7.7009) -> (-9.9335, -13.8009)
  line L228 (-9.9335, -13.8009) -> (-13.5816, -13.8009)
  line L229 (-13.5816, -13.8009) -> (-13.5816, -13.0792)
  spline S125 degree 2 poles (-16.7997, -8.1853) (-16.7058, -8.1161) (-16.3894, -7.8689) (-16.2411, -7.7948) knots 0 0 0 1 2 2 2
  spline S126 degree 2 poles (-16.2411, -7.7948) (-16.0385, -7.686) (-15.6578, -7.5724) (-15.3118, -7.5724) knots 0 0 0 1 2 2 2
  spline S127 degree 2 poles (-15.3118, -7.5724) (-15.03, -7.5724) (-14.5209, -7.7849) (-14.3281, -7.9777) knots 0 0 0 1 2 2 2
  spline S128 degree 2 poles (-14.3281, -7.9777) (-14.1452, -8.1655) (-13.9227, -8.7192) (-13.9227, -9.0257) knots 0 0 0 1 2 2 2
  spline S129 degree 2 poles (-13.9227, -9.0257) (-13.9227, -9.5002) (-14.3231, -10.1725) (-14.7581, -10.3653) knots 0 0 0 1 2 2 2
  spline S130 degree 2 poles (-14.7581, -10.3653) (-15.1437, -10.5433) (-16.1917, -10.6767) (-16.7997, -10.7113) knots 0 0 0 1 2 2 2
  line L230 (-16.7997, -10.7113) -> (-16.7997, -10.8596)
  spline S131 degree 2 poles (-16.7997, -10.8596) (-16.7997, -11.1266) (-16.6366, -11.4578) (-16.4883, -11.5517) knots 0 0 0 1 2 2 2
  spline S132 degree 2 poles (-16.4883, -11.5517) (-16.34, -11.6456) (-15.9149, -11.7049) (-15.6875, -11.7049) knots 0 0 0 1 2 2 2
  spline S133 degree 2 poles (-15.6875, -11.7049) (-15.4205, -11.7049) (-14.6988, -11.5467) (-14.338, -11.3935) knots 0 0 0 1 2 2 2
  line L231 (-14.338, -11.3935) -> (-14.2935, -11.3935)
  line L232 (-14.2935, -11.3935) -> (-14.2935, -12.1795)
  spline S134 degree 2 poles (-14.2935, -12.1795) (-14.506, -12.2388) (-15.3019, -12.3871) (-15.6924, -12.3871) knots 0 0 0 1 2 2 2
  spline S135 degree 2 poles (-15.6924, -12.3871) (-16.167, -12.3871) (-16.8145, -12.2388) (-17.0716, -12.046) knots 0 0 0 1 2 2 2
  spline S136 degree 2 poles (-17.0716, -12.046) (-17.3237, -11.8582) (-17.5709, -11.26) (-17.5709, -10.83) knots 0 0 0 1 2 2 2
  line L233 (-17.5709, -10.83) -> (-17.5709, -7.7009)
  line L234 (-17.5709, -7.7009) -> (-16.7997, -7.7009)
  line L235 (-16.7997, -7.7009) -> (-16.7997, -8.1853)
  line L236 (-16.7997, -8.8279) -> (-16.7997, -10.0984)
  spline S137 degree 2 poles (-16.7997, -10.0984) (-16.5229, -10.0736) (-15.6875, -9.9896) (-15.4255, -9.9105) knots 0 0 0 1 2 2 2
  spline S138 degree 2 poles (-15.4255, -9.9105) (-15.119, -9.8166) (-14.7186, -9.4261) (-14.7186, -9.0801) knots 0 0 0 1 2 2 2
  spline S139 degree 2 poles (-14.7186, -9.0801) (-14.7186, -8.6846) (-15.1635, -8.2842) (-15.5886, -8.2842) knots 0 0 0 1 2 2 2
  spline S140 degree 2 poles (-15.5886, -8.2842) (-15.9495, -8.2842) (-16.5427, -8.5956) (-16.7997, -8.8279) knots 0 0 0 1 2 2 2
  line L237 (-19.4394, -7.7009) -> (-18.6683, -7.7009)
  line L238 (-18.6683, -7.7009) -> (-18.6683, -14.0728)
  line L239 (-18.6683, -14.0728) -> (-19.4394, -14.0728)
  line L240 (-19.4394, -14.0728) -> (-19.4394, -7.7009)
  line L241 (-21.3574, -7.7009) -> (-20.5863, -7.7009)
  line L242 (-20.5863, -7.7009) -> (-20.5863, -12.2783)
  line L243 (-20.5863, -12.2783) -> (-21.3574, -12.2783)
  line L244 (-21.3574, -12.2783) -> (-21.3574, -7.7009)
  line L245 (-21.4118, -13.0396) -> (-20.5368, -13.0396)
  line L246 (-20.5368, -13.0396) -> (-20.5368, -13.8404)
  line L247 (-20.5368, -13.8404) -> (-21.4118, -13.8404)
  line L248 (-21.4118, -13.8404) -> (-21.4118, -13.0396)
  spline S141 degree 2 poles (-26.2513, -9.9896) (-26.2513, -8.8329) (-25.139, -7.5724) (-24.2097, -7.5724) knots 0 0 0 1 2 2 2
  spline S142 degree 2 poles (-24.2097, -7.5724) (-23.2556, -7.5724) (-22.1632, -8.8724) (-22.1632, -9.9896) knots 0 0 0 1 2 2 2
  spline S143 degree 2 poles (-22.1632, -9.9896) (-22.1632, -11.1365) (-23.2902, -12.4069) (-24.2097, -12.4069) knots 0 0 0 1 2 2 2
  spline S144 degree 2 poles (-24.2097, -12.4069) (-25.139, -12.4069) (-26.2513, -11.1414) (-26.2513, -9.9896) knots 0 0 0 1 2 2 2
  spline S145 degree 2 poles (-25.4554, -9.9896) (-25.4554, -10.8794) (-24.8078, -11.7445) (-24.2097, -11.7445) knots 0 0 0 1 2 2 2
  spline S146 degree 2 poles (-24.2097, -11.7445) (-23.6115, -11.7445) (-22.959, -10.8794) (-22.959, -9.9896) knots 0 0 0 1 2 2 2
  spline S147 degree 2 poles (-22.959, -9.9896) (-22.959, -9.1245) (-23.6115, -8.2348) (-24.2097, -8.2348) knots 0 0 0 1 2 2 2
  spline S148 degree 2 poles (-24.2097, -8.2348) (-24.8029, -8.2348) (-25.4554, -9.1097) (-25.4554, -9.9896) knots 0 0 0 1 2 2 2
  line L249 (-30.6359, -7.7009) -> (-29.8648, -7.7009)
  line L250 (-29.8648, -7.7009) -> (-29.8648, -10.3109)
  spline S149 degree 2 poles (-29.8648, -10.3109) (-29.8648, -10.6273) (-29.8055, -11.1711) (-29.7165, -11.3342) knots 0 0 0 1 2 2 2
  spline S150 degree 2 poles (-29.7165, -11.3342) (-29.6226, -11.5072) (-29.2864, -11.6753) (-28.9997, -11.6753) knots 0 0 0 1 2 2 2
  spline S151 degree 2 poles (-28.9997, -11.6753) (-28.713, -11.6753) (-28.105, -11.3688) (-27.8133, -11.1216) knots 0 0 0 1 2 2 2
  line L251 (-27.8133, -11.1216) -> (-27.8133, -7.7009)
  line L252 (-27.8133, -7.7009) -> (-27.0422, -7.7009)
  line L253 (-27.0422, -7.7009) -> (-27.0422, -12.2783)
  line L254 (-27.0422, -12.2783) -> (-27.8133, -12.2783)
  line L255 (-27.8133, -12.2783) -> (-27.8133, -11.7692)
  spline S152 degree 2 poles (-27.8133, -11.7692) (-28.1594, -12.0806) (-28.8267, -12.4069) (-29.2024, -12.4069) knots 0 0 0 1 2 2 2
  spline S153 degree 2 poles (-29.2024, -12.4069) (-29.8747, -12.4069) (-30.6359, -11.5171) (-30.6359, -10.6718) knots 0 0 0 1 2 2 2
  line L256 (-30.6359, -10.6718) -> (-30.6359, -7.7009)
  line L257 (32.5984, 2.3426) -> (32.5984, -3.7574)
  line L258 (32.5984, -3.7574) -> (28.7822, -3.7574)
  line L259 (28.7822, -3.7574) -> (28.7822, -3.0357)
  line L260 (28.7822, -3.0357) -> (31.7877, -3.0357)
  line L261 (31.7877, -3.0357) -> (31.7877, -1.3648)
  line L262 (31.7877, -1.3648) -> (28.9849, -1.3648)
  line L263 (28.9849, -1.3648) -> (28.9849, -0.6431)
  line L264 (28.9849, -0.6431) -> (31.7877, -0.6431)
  line L265 (31.7877, -0.6431) -> (31.7877, 1.6209)
  line L266 (31.7877, 1.6209) -> (28.7822, 1.6209)
  line L267 (28.7822, 1.6209) -> (28.7822, 2.3426)
  line L268 (28.7822, 2.3426) -> (32.5984, 2.3426)
  line L269 (24.358, 2.3426) -> (25.1291, 2.3426)
  line L270 (25.1291, 2.3426) -> (25.1291, -0.2674)
  spline S154 degree 2 poles (25.1291, -0.2674) (25.1291, -0.5838) (25.1885, -1.1276) (25.2774, -1.2907) knots 0 0 0 1 2 2 2
  spline S155 degree 2 poles (25.2774, -1.2907) (25.3714, -1.4637) (25.7075, -1.6318) (25.9942, -1.6318) knots 0 0 0 1 2 2 2
  spline S156 degree 2 poles (25.9942, -1.6318) (26.2809, -1.6318) (26.8889, -1.3253) (27.1806, -1.0781) knots 0 0 0 1 2 2 2
  line L271 (27.1806, -1.0781) -> (27.1806, 2.3426)
  line L272 (27.1806, 2.3426) -> (27.9517, 2.3426)
  line L273 (27.9517, 2.3426) -> (27.9517, -2.2349)
  line L274 (27.9517, -2.2349) -> (27.1806, -2.2349)
  line L275 (27.1806, -2.2349) -> (27.1806, -1.7257)
  spline S157 degree 2 poles (27.1806, -1.7257) (26.8346, -2.0371) (26.1672, -2.3634) (25.7915, -2.3634) knots 0 0 0 1 2 2 2
  spline S158 degree 2 poles (25.7915, -2.3634) (25.1192, -2.3634) (24.358, -1.4736) (24.358, -0.6283) knots 0 0 0 1 2 2 2
  line L276 (24.358, -0.6283) -> (24.358, 2.3426)
  spline S159 degree 2 poles (23.1123, 3.0742) (23.0332, 3.1088) (22.7316, 3.2176) (22.5389, 3.2621) knots 0 0 0 1 2 2 2
  spline S160 degree 2 poles (22.5389, 3.2621) (22.3263, 3.3164) (21.9654, 3.3807) (21.7529, 3.3807) knots 0 0 0 1 2 2 2
  spline S161 degree 2 poles (21.7529, 3.3807) (21.397, 3.3807) (20.9026, 3.1929) (20.7642, 3.0248) knots 0 0 0 1 2 2 2
  spline S162 degree 2 poles (20.7642, 3.0248) (20.6308, 2.8567) (20.5269, 2.4168) (20.5269, 2.135) knots 0 0 0 1 2 2 2
  line L277 (20.5269, 2.135) -> (20.5269, 1.7346)
  spline S163 degree 2 poles (20.5269, 1.7346) (20.8384, 2.0065) (21.4365, 2.2635) (21.8863, 2.2635) knots 0 0 0 1 2 2 2
  spline S164 degree 2 poles (21.8863, 2.2635) (22.6674, 2.2635) (23.5918, 1.1019) (23.5918, 0.0094) knots 0 0 0 1 2 2 2
  spline S165 degree 2 poles (23.5918, 0.0094) (23.5918, -0.5591) (23.2705, -1.439) (23.0035, -1.7504) knots 0 0 0 1 2 2 2
  spline S166 degree 2 poles (23.0035, -1.7504) (22.7465, -2.0421) (22.0396, -2.3634) (21.6639, -2.3634) knots 0 0 0 1 2 2 2
  spline S167 degree 2 poles (21.6639, -2.3634) (21.308, -2.3634) (20.7889, -2.1953) (20.5269, -2.0421) knots 0 0 0 1 2 2 2
  line L278 (20.5269, -2.0421) -> (20.4825, -2.2349)
  line L279 (20.4825, -2.2349) -> (19.7558, -2.2349)
  line L280 (19.7558, -2.2349) -> (19.7558, 1.8186)
  spline S168 degree 2 poles (19.7558, 1.8186) (19.7558, 2.9852) (20.7692, 4.0728) (21.8122, 4.0728) knots 0 0 0 1 2 2 2
  spline S169 degree 2 poles (21.8122, 4.0728) (22.1483, 4.0728) (22.8503, 3.964) (23.1518, 3.875) knots 0 0 0 1 2 2 2
  line L281 (23.1518, 3.875) -> (23.1518, 3.0742)
  line L282 (23.1518, 3.0742) -> (23.1123, 3.0742)
  line L283 (20.5269, 1.1019) -> (20.5269, -1.4143)
  spline S170 degree 2 poles (20.5269, -1.4143) (20.8137, -1.5527) (21.2981, -1.6713) (21.5403, -1.6713) knots 0 0 0 1 2 2 2
  spline S171 degree 2 poles (21.5403, -1.6713) (22.1236, -1.6713) (22.7959, -0.8112) (22.7959, -0.0054) knots 0 0 0 1 2 2 2
  spline S172 degree 2 poles (22.7959, -0.0054) (22.7959, 0.7558) (22.2867, 1.5517) (21.7133, 1.5517) knots 0 0 0 1 2 2 2
  spline S173 degree 2 poles (21.7133, 1.5517) (21.4118, 1.5517) (20.7791, 1.3144) (20.5269, 1.1019) knots 0 0 0 1 2 2 2
  line L284 (17.4423, 2.3426) -> (18.4211, 2.3426)
  line L285 (18.4211, 2.3426) -> (18.4211, 1.176)
  line L286 (18.4211, 1.176) -> (17.4423, 1.176)
  line L287 (17.4423, 1.176) -> (17.4423, 2.3426)
  line L288 (14.076, 2.3426) -> (12.0196, -3.7574)
  line L289 (12.0196, -3.7574) -> (11.021, -3.7574)
  line L290 (11.021, -3.7574) -> (8.9646, 2.3426)
  line L291 (8.9646, 2.3426) -> (9.8198, 2.3426)
  line L292 (9.8198, 2.3426) -> (10.3735, 0.6372)
  line L293 (10.3735, 0.6372) -> (12.7017, 0.6372)
  line L294 (12.7017, 0.6372) -> (13.2554, 2.3426)
  line L295 (13.2554, 2.3426) -> (14.076, 2.3426)
  line L296 (10.5959, -0.0549) -> (11.5401, -2.9269)
  line L297 (11.5401, -2.9269) -> (12.4793, -0.0549)
  line L298 (12.4793, -0.0549) -> (10.5959, -0.0549)
  line L299 (7.6596, 2.3426) -> (8.4308, 2.3426)
  line L300 (8.4308, 2.3426) -> (8.4308, -4.0293)
  line L301 (8.4308, -4.0293) -> (7.6596, -4.0293)
  line L302 (7.6596, -4.0293) -> (7.6596, 2.3426)
  line L303 (5.7416, 2.3426) -> (6.5128, 2.3426)
  line L304 (6.5128, 2.3426) -> (6.5128, -2.2349)
  line L305 (6.5128, -2.2349) -> (5.7416, -2.2349)
  line L306 (5.7416, -2.2349) -> (5.7416, 2.3426)
  line L307 (5.6872, -2.9961) -> (6.5622, -2.9961)
  line L308 (6.5622, -2.9961) -> (6.5622, -3.7969)
  line L309 (6.5622, -3.7969) -> (5.6872, -3.7969)
  line L310 (5.6872, -3.7969) -> (5.6872, -2.9961)
  line L311 (2.5878, 2.3426) -> (0.5314, -3.7574)
  line L312 (0.5314, -3.7574) -> (-0.4671, -3.7574)
  line L313 (-0.4671, -3.7574) -> (-2.5235, 2.3426)
  line L314 (-2.5235, 2.3426) -> (-1.6684, 2.3426)
  line L315 (-1.6684, 2.3426) -> (-1.1147, 0.6372)
  line L316 (-1.1147, 0.6372) -> (1.2136, 0.6372)
  line L317 (1.2136, 0.6372) -> (1.7672, 2.3426)
  line L318 (1.7672, 2.3426) -> (2.5878, 2.3426)
  line L319 (-0.8923, -0.0549) -> (0.0519, -2.9269)
  line L320 (0.0519, -2.9269) -> (0.9911, -0.0549)
  line L321 (0.9911, -0.0549) -> (-0.8923, -0.0549)
  line L322 (-3.8286, 2.3426) -> (-3.0574, 2.3426)
  line L323 (-3.0574, 2.3426) -> (-3.0574, -4.0293)
  line L324 (-3.0574, -4.0293) -> (-3.8286, -4.0293)
  line L325 (-3.8286, -4.0293) -> (-3.8286, 2.3426)
  line L326 (-6.9824, 2.3426) -> (-9.0388, -3.7574)
  line L327 (-9.0388, -3.7574) -> (-10.0373, -3.7574)
  line L328 (-10.0373, -3.7574) -> (-12.0937, 2.3426)
  line L329 (-12.0937, 2.3426) -> (-11.2385, 2.3426)
  line L330 (-11.2385, 2.3426) -> (-10.6849, 0.6372)
  line L331 (-10.6849, 0.6372) -> (-8.3566, 0.6372)
  line L332 (-8.3566, 0.6372) -> (-7.803, 2.3426)
  line L333 (-7.803, 2.3426) -> (-6.9824, 2.3426)
  line L334 (-10.4624, -0.0549) -> (-9.5183, -2.9269)
  line L335 (-9.5183, -2.9269) -> (-8.5791, -0.0549)
  line L336 (-8.5791, -0.0549) -> (-10.4624, -0.0549)
  spline S174 degree 2 poles (-16.4487, -0.0203) (-16.4487, 1.1019) (-15.3612, 2.4711) (-14.5406, 2.4711) knots 0 0 0 1 2 2 2
  spline S175 degree 2 poles (-14.5406, 2.4711) (-14.1699, 2.4711) (-13.641, 2.2882) (-13.3839, 2.1301) knots 0 0 0 1 2 2 2
  line L337 (-13.3839, 2.1301) -> (-13.3345, 2.3426)
  line L338 (-13.3345, 2.3426) -> (-12.6128, 2.3426)
  line L339 (-12.6128, 2.3426) -> (-12.6128, -4.0293)
  line L340 (-12.6128, -4.0293) -> (-13.3839, -4.0293)
  line L341 (-13.3839, -4.0293) -> (-13.3839, -1.7554)
  spline S176 degree 2 poles (-13.3839, -1.7554) (-13.6756, -2.0174) (-14.3528, -2.3634) (-14.7829, -2.3634) knots 0 0 0 1 2 2 2
  spline S177 degree 2 poles (-14.7829, -2.3634) (-15.559, -2.3634) (-16.4487, -1.1226) (-16.4487, -0.0203) knots 0 0 0 1 2 2 2
  spline S178 degree 2 poles (-15.6529, 0.039) (-15.6529, -0.7815) (-15.1536, -1.6318) (-14.6, -1.6318) knots 0 0 0 1 2 2 2
  spline S179 degree 2 poles (-14.6, -1.6318) (-14.2885, -1.6318) (-13.6459, -1.3352) (-13.3839, -1.1078) knots 0 0 0 1 2 2 2
  line L342 (-13.3839, -1.1078) -> (-13.3839, 1.5171)
  spline S180 degree 2 poles (-13.3839, 1.5171) (-13.6756, 1.6604) (-14.1254, 1.7791) (-14.3923, 1.7791) knots 0 0 0 1 2 2 2
  spline S181 degree 2 poles (-14.3923, 1.7791) (-14.9806, 1.7791) (-15.6529, 0.9437) (-15.6529, 0.039) knots 0 0 0 1 2 2 2
  spline S182 degree 2 poles (-21.0855, -0.0203) (-21.0855, 1.1019) (-19.998, 2.4711) (-19.1774, 2.4711) knots 0 0 0 1 2 2 2
  spline S183 degree 2 poles (-19.1774, 2.4711) (-18.8067, 2.4711) (-18.2778, 2.2882) (-18.0207, 2.1301) knots 0 0 0 1 2 2 2
  line L343 (-18.0207, 2.1301) -> (-17.9713, 2.3426)
  line L344 (-17.9713, 2.3426) -> (-17.2496, 2.3426)
  line L345 (-17.2496, 2.3426) -> (-17.2496, -4.0293)
  line L346 (-17.2496, -4.0293) -> (-18.0207, -4.0293)
  line L347 (-18.0207, -4.0293) -> (-18.0207, -1.7554)
  spline S184 degree 2 poles (-18.0207, -1.7554) (-18.3124, -2.0174) (-18.9896, -2.3634) (-19.4197, -2.3634) knots 0 0 0 1 2 2 2
  spline S185 degree 2 poles (-19.4197, -2.3634) (-20.1957, -2.3634) (-21.0855, -1.1226) (-21.0855, -0.0203) knots 0 0 0 1 2 2 2
  spline S186 degree 2 poles (-20.2897, 0.039) (-20.2897, -0.7815) (-19.7904, -1.6318) (-19.2368, -1.6318) knots 0 0 0 1 2 2 2
  spline S187 degree 2 poles (-19.2368, -1.6318) (-18.9253, -1.6318) (-18.2827, -1.3352) (-18.0207, -1.1078) knots 0 0 0 1 2 2 2
  line L348 (-18.0207, -1.1078) -> (-18.0207, 1.5171)
  spline S188 degree 2 poles (-18.0207, 1.5171) (-18.3124, 1.6604) (-18.7622, 1.7791) (-19.0291, 1.7791) knots 0 0 0 1 2 2 2
  spline S189 degree 2 poles (-19.0291, 1.7791) (-19.6174, 1.7791) (-20.2897, 0.9437) (-20.2897, 0.039) knots 0 0 0 1 2 2 2
  spline S190 degree 2 poles (-24.4371, 1.8582) (-24.3432, 1.9274) (-24.0268, 2.1745) (-23.8785, 2.2487) knots 0 0 0 1 2 2 2
  spline S191 degree 2 poles (-23.8785, 2.2487) (-23.6758, 2.3574) (-23.2952, 2.4711) (-22.9492, 2.4711) knots 0 0 0 1 2 2 2
  spline S192 degree 2 poles (-22.9492, 2.4711) (-22.6674, 2.4711) (-22.1582, 2.2586) (-21.9654, 2.0658) knots 0 0 0 1 2 2 2
  spline S193 degree 2 poles (-21.9654, 2.0658) (-21.7825, 1.8779) (-21.5601, 1.3243) (-21.5601, 1.0178) knots 0 0 0 1 2 2 2
  spline S194 degree 2 poles (-21.5601, 1.0178) (-21.5601, 0.5433) (-21.9605, -0.129) (-22.3955, -0.3218) knots 0 0 0 1 2 2 2
  spline S195 degree 2 poles (-22.3955, -0.3218) (-22.7811, -0.4998) (-23.8291, -0.6332) (-24.4371, -0.6678) knots 0 0 0 1 2 2 2
  line L349 (-24.4371, -0.6678) -> (-24.4371, -0.8161)
  spline S196 degree 2 poles (-24.4371, -0.8161) (-24.4371, -1.0831) (-24.2739, -1.4143) (-24.1257, -1.5082) knots 0 0 0 1 2 2 2
  spline S197 degree 2 poles (-24.1257, -1.5082) (-23.9774, -1.6021) (-23.5522, -1.6614) (-23.3248, -1.6614) knots 0 0 0 1 2 2 2
  spline S198 degree 2 poles (-23.3248, -1.6614) (-23.0579, -1.6614) (-22.3362, -1.5033) (-21.9753, -1.35) knots 0 0 0 1 2 2 2
  line L350 (-21.9753, -1.35) -> (-21.9308, -1.35)
  line L351 (-21.9308, -1.35) -> (-21.9308, -2.136)
  spline S199 degree 2 poles (-21.9308, -2.136) (-22.1434, -2.1953) (-22.9393, -2.3436) (-23.3298, -2.3436) knots 0 0 0 1 2 2 2
  spline S200 degree 2 poles (-23.3298, -2.3436) (-23.8043, -2.3436) (-24.4519, -2.1953) (-24.709, -2.0025) knots 0 0 0 1 2 2 2
  spline S201 degree 2 poles (-24.709, -2.0025) (-24.9611, -1.8147) (-25.2082, -1.2165) (-25.2082, -0.7865) knots 0 0 0 1 2 2 2
  line L352 (-25.2082, -0.7865) -> (-25.2082, 2.3426)
  line L353 (-25.2082, 2.3426) -> (-24.4371, 2.3426)
  line L354 (-24.4371, 2.3426) -> (-24.4371, 1.8582)
  line L355 (-24.4371, 1.2155) -> (-24.4371, -0.0549)
  spline S202 degree 2 poles (-24.4371, -0.0549) (-24.1603, -0.0302) (-23.3248, 0.0539) (-23.0628, 0.133) knots 0 0 0 1 2 2 2
  spline S203 degree 2 poles (-23.0628, 0.133) (-22.7564, 0.2269) (-22.356, 0.6174) (-22.356, 0.9634) knots 0 0 0 1 2 2 2
  spline S204 degree 2 poles (-22.356, 0.9634) (-22.356, 1.3589) (-22.8009, 1.7593) (-23.226, 1.7593) knots 0 0 0 1 2 2 2
  spline S205 degree 2 poles (-23.226, 1.7593) (-23.5868, 1.7593) (-24.18, 1.4479) (-24.4371, 1.2155) knots 0 0 0 1 2 2 2
  spline S206 degree 2 poles (-27.5266, 2.4514) (-27.0669, 2.4514) (-26.271, 2.2042) (-26.009, 2.0658) knots 0 0 0 1 2 2 2
  line L356 (-26.009, 2.0658) -> (-26.009, 1.2007)
  line L357 (-26.009, 1.2007) -> (-26.0486, 1.2007)
  spline S207 degree 2 poles (-26.0486, 1.2007) (-26.1474, 1.2798) (-26.4144, 1.4677) (-26.6368, 1.5715) knots 0 0 0 1 2 2 2
  spline S208 degree 2 poles (-26.6368, 1.5715) (-26.8296, 1.6654) (-27.3042, 1.8038) (-27.5563, 1.8038) knots 0 0 0 1 2 2 2
  spline S209 degree 2 poles (-27.5563, 1.8038) (-27.7392, 1.8038) (-28.1594, 1.7198) (-28.2582, 1.6506) knots 0 0 0 1 2 2 2
  spline S210 degree 2 poles (-28.2582, 1.6506) (-28.4016, 1.5566) (-28.5301, 1.3441) (-28.5301, 1.1266) knots 0 0 0 1 2 2 2
  spline S211 degree 2 poles (-28.5301, 1.1266) (-28.5301, 0.8547) (-28.2335, 0.5729) (-27.8529, 0.479) knots 0 0 0 1 2 2 2
  spline S212 degree 2 poles (-27.8529, 0.479) (-27.7046, 0.4444) (-27.23, 0.3455) (-27.0274, 0.2912) knots 0 0 0 1 2 2 2
  spline S213 degree 2 poles (-27.0274, 0.2912) (-26.5034, 0.1379) (-26.0288, -0.4948) (-26.0288, -0.9447) knots 0 0 0 1 2 2 2
  spline S214 degree 2 poles (-26.0288, -0.9447) (-26.0288, -1.5675) (-26.9631, -2.3436) (-27.7342, -2.3436) knots 0 0 0 1 2 2 2
  spline S215 degree 2 poles (-27.7342, -2.3436) (-28.1149, -2.3436) (-28.886, -2.1558) (-29.148, -2.0124) knots 0 0 0 1 2 2 2
  line L358 (-29.148, -2.0124) -> (-29.148, -1.1869)
  line L359 (-29.148, -1.1869) -> (-29.1085, -1.1869)
  spline S216 degree 2 poles (-29.1085, -1.1869) (-28.8119, -1.4242) (-28.0902, -1.696) (-27.7194, -1.696) knots 0 0 0 1 2 2 2
  spline S217 degree 2 poles (-27.7194, -1.696) (-27.3388, -1.696) (-26.8148, -1.3747) (-26.8148, -1.0534) knots 0 0 0 1 2 2 2
  spline S218 degree 2 poles (-26.8148, -1.0534) (-26.8148, -0.7618) (-27.1262, -0.48) (-27.4722, -0.391) knots 0 0 0 1 2 2 2
  spline S219 degree 2 poles (-27.4722, -0.391) (-27.6403, -0.3465) (-28.0654, -0.2575) (-28.2978, -0.2032) knots 0 0 0 1 2 2 2
  spline S220 degree 2 poles (-28.2978, -0.2032) (-28.802, -0.0746) (-29.3161, 0.5136) (-29.3161, 1.0228) knots 0 0 0 1 2 2 2